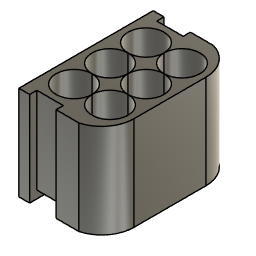
bottom weight batteries (Autodesk Fusion 360 design; units mm, degrees)
Autodesk Fusion 360 part; units mm, degrees
sketch "Esquisse1" plane through (0, 0, 0) normal (0, 0, 1) x (1, 0, 0)
  circle A0 centre (0, 0) radius 7.5
  circle A1 centre (0, 15) radius 7.5
  circle A2 centre (0, -15) radius 7.5
  circle A3 centre (15, 0) radius 7.5
  circle A4 centre (15, -15) radius 7.5
  circle A5 centre (15, 15) radius 7.5
  line L0 (25, 16) -> (25, -16)
  line L1 (5.5, 25) -> (-5.5, 25)
  line L2 (5.5, -25) -> (-5.5, -25)
  line L3 (-10, 25) -> (-10, -25)
  line L4 (-5.5, 25) -> (5.5, 25)
  line L5 (-10, 28) -> (-10, 25)
  line L6 (0, 25) -> (-5.5, 25)
  line L7 (-5.5, 25) -> (5.5, 25)
  line L8 (5.5, 25) -> (5.5, 28)
  line L9 (-5.5, 28) -> (-5.5, 25)
  line L10 (15, 28) -> (5.5, 28)
  line L11 (-5.5, 28) -> (-10, 28)
  line L12 (25, 0) -> (22.5, 0)
  line L13 (15, -28) -> (5.5, -28)
  line L14 (5.5, -25) -> (5.5, -28)
  line L15 (-5.5, -25) -> (5.5, -25)
  line L16 (-5.5, -28) -> (-5.5, -25)
  line L17 (-5.5, -28) -> (-10, -28)
  line L18 (-10, -28) -> (-10, -25)
  line L19 (15, -15) -> (25, -15)
  line L20 (15, -15) -> (15, -28)
  arc A6 (15, -28) -> (25, -15) centre (11.55, -15) ccw
  line L21 (15, 15) -> (15, 28)
  line L22 (15, 15) -> (25, 15)
  arc A7 (25, 15) -> (15, 28) centre (11.55, 15) ccw
  line L23 (-5.5, 25) -> (5.5, 25)
  line L24 (5.5, 25) -> (5.5, -25)
  line L25 (5.5, -25) -> (-5.5, -25)
  line L26 (-5.5, -25) -> (-5.5, 25)
  dimension "d1" = 15
  dimension "d17" = 15
  dimension "d21" = 360
  dimension "d23" = 360
  dimension "d40" = 3
  dimension "d41" = 5.5
  dimension "d42" = 11
  constraint coincident A0.centre origin
  constraint tangent A0 A1
  constraint vertical L0
  constraint perpendicular L2 L3
  constraint horizontal L4
  constraint horizontal L10
  constraint vertical L5
  constraint coincident L1 L6.start
  constraint horizontal L7
  constraint vertical L8
  constraint vertical L9
  constraint collinear L10 L11
  constraint midpoint L0 L12.start
  constraint coincident A3 L12.end
  constraint perpendicular L0 L12
  constraint symmetric L3.start L12 L3.end
  constraint symmetric L5.start L12 L17.end
  constraint symmetric L1.end L12 L2.end
  constraint symmetric L1.start L12 L2.start
  constraint symmetric L8.end L12 L13.end
  constraint symmetric L9.start L12 L16.start
  constraint coincident A4.centre L19.start
  constraint coincident L0 L19.end
  constraint perpendicular L0 L19
  constraint perpendicular L13 L20
  constraint coincident A5.centre L21.start
  constraint perpendicular L10 L21
  constraint coincident L0 L22.end
  constraint perpendicular L0 L22
  constraint tangent L0 A7
  constraint horizontal L23
  constraint vertical L24
  constraint horizontal L25
  constraint vertical L26
  measures "d1" diameter of A0
  measures "d17" distance of A0.centre A1.centre
  measures "d40" distance of L3.start L5.start
  measures "d41" distance of L6.start L1.end
  measures "d42" distance of L1.end L1.start
extrude "Extrusion7" add sketch "Esquisse1" against normal blind 4.2 contours A0 L24 | A0 A2 A3 A4 L24 | A0 A1 A3 A5 L24 | A3 | A3 A5 L0 L12 L22 | A5 L21 L22 | A3 A4 L0 L12 L19 | A4 L19 L20 | A1 L24 | A2 L24 | A1 A5 L8 L10 L21 L24 | A5 L21 L22 | A5 L21 L22 A7 | A4 L19 L20 A6 | A4 L19 L20 | A2 A4 L13 L14 L20 L24 | A0 L26 | A0 A1 A2 L3 L5 L9 L11 L16 L17 L18 L26 | A1 L26 | A2 L26 makes body 1 at (-7, -9.3333, 0) makes body 2 at (12, 5, 0)
extrude "Extrusion8" add sketch "Esquisse1" against normal blind 1 bodies 1 2
extrude "Extrusion9" add sketch "Esquisse1" along normal blind 35 contours A0 A2 A3 A4 L24 | A0 A1 A3 A5 L24 | A0 A1 L24 | A0 A2 L24 | A3 A5 L0 L12 L22 | A3 A4 L0 L12 L19 | A0 A1 L26 | A0 A2 L26 | A1 A5 L8 L10 L21 L24 | A5 L21 L22 A7 | A4 L19 L20 A6 | A2 A4 L13 L14 L20 L24 | A0 A1 A2 L3 L5 L9 L11 L16 L17 L18 L26 | A1 L1 L4 L6 L7 L23 L24 L26 | A2 L2 L15 L24 L25 L26 bodies 1
